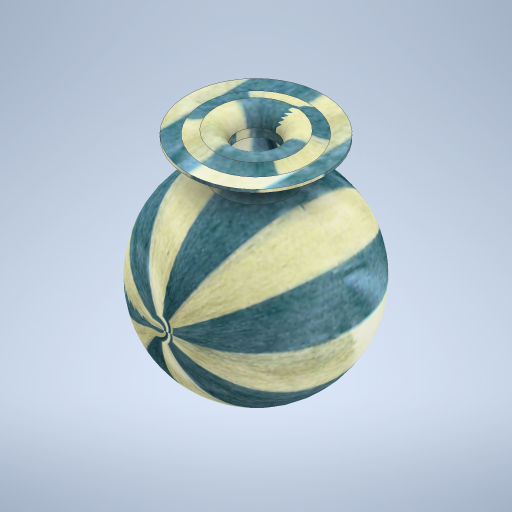
# Autodesk Inventor part: Versaball membrane
Saved by Autodesk Inventor 2023 (Build 270158030, 158C)
## iProperties
Created: 2022-09-15
Part Number: Versaball membrane
Material: Canvas, Blue Stripe
Document SubType Name: Modeling
Designer: cjj5381
Density: 0.152 g/cm^3
Appearance: Stripes - Blue-White
Author: cjj5381
Autodesk Inventor part; units mm, degrees
ref_plane "YZ Plane" through (0, 0, 0) normal (1, 0, 0) x (0, 1, 0)
ref_plane "XZ Plane" through (0, 0, 0) normal (0, 1, 0) x (-1, 0, 0)
ref_plane "XY Plane" through (0, 0, 0) normal (0, 0, 1) x (1, 0, 0)
sketch "Sketch1" plane through (0, 0, 0) normal (0, 0, 1) x (1, 0, 0)
  arc A0 (0, -76.2) -> (29.0763, 70.4344) centre (0, 0) ccw
  arc A1 (16.51, 89.2169) -> (29.0763, 70.4344) centre (36.83, 89.2169) ccw
  line L0 (0, 0) -> (0, 160.2867)
  line L1 (0, 0) -> (0, -138.0846)
  line L2 (0, -74.93) -> (0, -76.2)
  line L3 (16.51, 89.2169) -> (16.51, 95.9932)
  arc A2 (33.4433, 106.0111) -> (16.51, 95.9932) centre (27.94, 95.9932) ccw
  arc A3 (33.4433, 106.0111) -> (44.45, 103.1869) centre (44.45, 126.0469) ccw
  line L4 (44.45, 103.1869) -> (57.15, 103.1869)
  arc A4 (0, -78.74) -> (30.0455, 72.7822) centre (0, 0) ccw
  arc A5 (19.05, 89.2169) -> (30.0455, 72.7822) centre (36.83, 89.2169) ccw
  line L5 (19.05, 89.2169) -> (19.05, 95.9932)
  arc A6 (32.2204, 103.7849) -> (19.05, 95.9932) centre (27.94, 95.9932) ccw
  arc A7 (32.2204, 103.7849) -> (44.45, 100.6469) centre (44.45, 126.0469) ccw
  line L6 (44.45, 100.6469) -> (57.15, 100.6469)
  line L7 (57.15, 103.1869) -> (57.15, 100.6469)
  line L8 (0, -76.2) -> (0, -78.74)
  dimension "d0" = 152.4
  dimension "d8" = 114.3
  dimension "d9" = 22.86
  dimension "d10" = 2.54
  dimension "d11" = 78.74
  dimension "d13" = 25.4
  dimension "d14" = 11.43
  dimension "d15" = 17.78
  dimension "d16" = 38.1
  dimension "d18" = 88.9
  constraints: 18 end point, 16 point on circle, 8 centre point, 5 tangent, 4 vertical, 2 point on line, 1 coincident, 1 collinear, 1 horizontal, 4 other
  measures "d0" diameter of A0
  measures "d8" diameter of L4.end L0
  measures "d9" diameter of A2
  measures "d10" radial gap between concentric circles of A1 A5
  measures "d11" radius of A4
  measures "d13" radius of A7
  measures "d14" distance from line of A1.centre L6
  measures "d15" radius of A5
  measures "d16" diameter of L5 L0
  measures "d18" diameter of A3.centre L0
revolve "Revolution1" add sketch "Sketch1" angle 360 about axis through (0, 0, 0) along (0, 1, 0)
body "Solid1"
